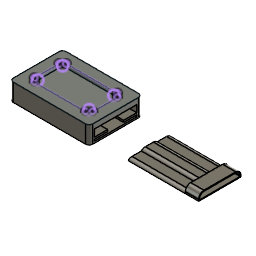
PRJCT (Autodesk Fusion 360 design; units mm, degrees)
part number: 2026-03-16-23-07-20-677
Autodesk Fusion 360 part; units mm, degrees
sketch "Esquisse1" plane through (0, 0, 0) normal (0, 1, 0) x (1, 0, 0)
  line L0 (22.5, 15) -> (-22.5, 15)
  line L1 (-22.5, 15) -> (-22.5, -15)
  line L2 (-22.5, -15) -> (22.5, -15)
  line L3 (22.5, -15) -> (22.5, 15)
  line L4 (22.5, 15) -> (-22.5, -15) construction
  line L5 (-22.5, 15) -> (22.5, -15) construction
  dimension "d1" = 30
  dimension "d2" = 45
  constraint horizontal L0
  constraint perpendicular L0 L1
  constraint parallel L0 L2
  constraint parallel L1 L3
  constraint coincident L4 origin
  constraint coincident L5 origin
  measures "d1" distance of L0.start L2.end
  measures "d2" distance of L0.start L0.end
extrude "Extrusion1" add sketch "Esquisse1" along normal blind 10 makes body 1
sketch "Esquisse2" plane through (22.5, 0, 0) normal (1, 0, 0) x (0, 0, -1)
  line L0 (-15, 0) -> (15, 0)
  line L1 (15, 0) -> (15, 10)
  line L2 (15, 10) -> (-15, 10)
  line L3 (-15, 10) -> (-15, 0)
  line L4 (-12, 7) -> (12, 7)
  line L5 (12, 7) -> (12, 3)
  line L6 (12, 3) -> (-12, 3)
  line L7 (-12, 3) -> (-12, 7)
  constraint horizontal L4
  constraint vertical L5
  constraint horizontal L6
  constraint vertical L7
sketch "Esquisse4" plane through (0, 10, 0) normal (0, 1, 0) x (-1, 0, 0)
  line L0 (-22.5, 15) -> (-22.5, -15)
  line L1 (-22.5, -15) -> (22.5, -15)
  line L2 (22.5, -15) -> (22.5, 15)
  line L3 (22.5, 15) -> (-22.5, 15)
  line L4 (16.5, 9) -> (-16.5, 9)
  line L5 (-16.5, 9) -> (-16.5, -9)
  line L6 (-16.5, -9) -> (16.5, -9)
  line L7 (16.5, -9) -> (16.5, 9)
  line L8 (16.5, 9) -> (-16.5, -9) construction
  line L9 (-16.5, 9) -> (16.5, -9) construction
  dimension "d9" = 6
  dimension "d10" = 6
  constraint horizontal L4
  constraint perpendicular L4 L5
  constraint parallel L4 L6
  constraint parallel L5 L7
  constraint coincident L8 origin
  constraint coincident L9 origin
  measures "d9" distance of L3 L4
  measures "d10" distance of L0 L5
extrude "Extrusion3" cut sketch "Esquisse4" against normal blind 2 contours L4 L5 L6 L7 bodies 1
fillet "Congé2" radius 2 4 edges at (-16.5, 9, -9) (-16.5, 9, 9) (16.5, 9, 9) (16.5, 9, -9) on bodies 1
extrude "Extrusion2" cut sketch "Esquisse2" against normal blind 40 contours L4 L5 L6 L7 bodies 1
fillet "Congé1" radius 2 4 edges at (22.5, 5, 15) (-22.5, 5, 15) (22.5, 5, -15) (-22.5, 5, -15) on bodies 1
sketch "Esquisse3" plane through (0, 10, 0) normal (0, 1, 0) x (-1, 0, 0)
  arc A0 (20.5, -15) -> (22.5, -13) centre (20.5, -13) ccw
  line L0 (22.5, -13) -> (22.5, 13)
  arc A1 (22.5, 13) -> (20.5, 15) centre (20.5, 13) ccw
  line L1 (20.5, 15) -> (-20.5, 15)
  arc A2 (-20.5, 15) -> (-22.5, 13) centre (-20.5, 13) ccw
  line L2 (-22.5, 13) -> (-22.5, -13)
  arc A3 (-22.5, -13) -> (-20.5, -15) centre (-20.5, -13) ccw
  line L3 (-20.5, -15) -> (20.5, -15)
  line L4 (-14.5, 9) -> (14.5, 9)
  arc A4 (16.5, 7) -> (14.5, 9) centre (14.5, 7) ccw
  line L5 (16.5, 7) -> (16.5, -7)
  arc A5 (14.5, -9) -> (16.5, -7) centre (14.5, -7) ccw
  line L6 (14.5, -9) -> (-14.5, -9)
  arc A6 (-16.5, -7) -> (-14.5, -9) centre (-14.5, -7) ccw
  line L7 (-16.5, -7) -> (-16.5, 7)
  arc A7 (-14.5, 9) -> (-16.5, 7) centre (-14.5, 7) ccw
sketch "Esquisse5" plane through (22.5, 0, 0) normal (1, 0, 0) x (0, 0, -1)
  line L0 (12, 7) -> (12, 3)
  line L1 (12, 3) -> (-12, 3)
  line L2 (-12, 3) -> (-12, 7)
  line L3 (-12, 7) -> (12, 7)
  line L4 (13, 0) -> (13, 10)
  line L5 (13, 10) -> (-13, 10)
  line L6 (-13, 10) -> (-13, 0)
  line L7 (-13, 0) -> (13, 0)
  line L8 (-4.5, 3) -> (4.5, 3)
  line L9 (4.5, 3) -> (4.5, 2)
  line L10 (4.5, 2) -> (-4.5, 2)
  line L11 (-4.5, 2) -> (-4.5, 3)
  line L12 (-12, 2) -> (12, 2)
  line L13 (12, 2) -> (12, 1)
  line L14 (12, 1) -> (-12, 1)
  line L15 (-12, 1) -> (-12, 2)
  dimension "d15" = 7.5
  dimension "d16" = 7.5
  constraint horizontal L8
  constraint vertical L9
  constraint horizontal L10
  constraint vertical L11
  constraint coincident L1 L8.start
  constraint horizontal L12
  constraint vertical L13
  constraint horizontal L14
  constraint vertical L15
  measures "d15" distance of L2 L11
  measures "d16" distance of L0 L9
extrude "Extrusion4" cut sketch "Esquisse5" against normal blind 24 contours L1 L8 L9 L10 L11 L12 | L10 L12 L13 L14 L15 bodies 1
extrude "Extrusion5" add 1 faces at (-1.5, 1.3333, 1.5) along direction (1, 0, 0) blind 40 separate body on bodies 1 makes body 2
move_body "Déplacer1" bodies 2 to x (1, 0, 0) y (0, 1, 0) z (0, 0, 1) at (43, 0, 0)
sketch "Esquisse6" plane through (0, 2, 0) normal (0, 1, 0) x (-1, 0, 0)
  line L0 (-41.5, 4.5) -> (-41.5, 12)
  line L1 (-41.5, 12) -> (-81.5, 12)
  line L2 (-81.5, 12) -> (-81.5, 4.5)
  line L3 (-81.5, 4.5) -> (-41.5, 4.5)
  line L4 (-81.5, 12) -> (-91, 12)
  line L5 (-91, 12) -> (-91, -12)
  line L6 (-91, -12) -> (-81.5, -12)
  line L7 (-81.5, -12) -> (-81.5, 12)
  constraint horizontal L4
  constraint vertical L5
  constraint horizontal L6
  constraint vertical L7
  constraint coincident L1.end L2.start
sketch "Esquisse7" plane through (0, 2, 0) normal (0, 1, 0) x (-1, 0, 0)
  line L0 (-41.5, 4.5) -> (-41.5, 12)
  line L1 (-41.5, 12) -> (-81.5, 12)
  line L2 (-81.5, 12) -> (-81.5, 4.5)
  line L3 (-81.5, 4.5) -> (-41.5, 4.5)
  line L4 (-81.5, 12) -> (-74, 12)
  line L5 (-74, 12) -> (-74, -12)
  line L6 (-74, -12) -> (-81.5, -12)
  line L7 (-81.5, -12) -> (-81.5, 12)
  constraint horizontal L4
  constraint vertical L5
  constraint horizontal L6
  constraint vertical L7
  constraint coincident L1.end L2.start
extrude "Extrusion7" add sketch "Esquisse7" along normal blind 3 contours L3 L5 L6 L7 | L1 L2 L3 L4 L5 L7 bodies 2
fillet "Congé5" radius 3 6 edges at (77.75, 5, -12) (77.75, 5, 12) (57.75, 3, -4.5) (57.75, 2, -12) (57.75, 2, 12) (57.75, 3, 4.5) on bodies 2
shell "Coque2" thickness 0.5 removed faces 1 at (81.5, 2.3333, -3) on bodies 2
